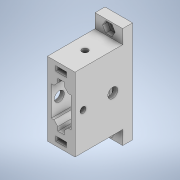
# Autodesk Inventor part: стаканчик_мозговорот
Saved by Autodesk Inventor 2021 (Build 250183000, 183)
## iProperties
Created: 2022-11-16
Part Number: стаканчик_мозговорот
Material: Типовые
Document SubType Name: Modeling
Designer: zmoze
Density: 1 g/cm^3
Appearance: По умолчанию
Author: zmoze
Autodesk Inventor part; units mm, degrees
sketch "Эскиз1" plane through (0, 0, 0) normal (0, 0, 1) x (1, 0, 0)
  line L0 (0, 0) -> (3.3, 0)
  line L1 (3.3, 0) -> (3.3, 15)
  line L2 (3.3, 15) -> (0, 15)
  line L3 (0, 15) -> (0, 0)
  line L4 (3.3, -4) -> (6.6, -4)
  line L5 (6.6, -4) -> (6.6, 19)
  line L6 (6.6, 19) -> (3.3, 19)
  line L7 (3.3, 19) -> (3.3, -4)
  line L8 (6.6, 0) -> (9.9, 0)
  line L9 (9.9, 0) -> (9.9, 15)
  line L10 (9.9, 15) -> (6.6, 15)
  line L11 (6.6, 15) -> (6.6, 0)
  line L12 (-2, 21) -> (11.9, 21)
  line L13 (11.9, 21) -> (11.9, -6)
  line L14 (11.9, -6) -> (-2, -6)
  line L15 (-2, -6) -> (-2, 21)
  dimension "d2" = 15
  dimension "d3" = 23
  dimension "d4" = 4
  dimension "d5" = 3.3
  dimension "d6" = 2
  dimension "d7" = 2
  dimension "d8" = 2
  dimension "d9" = 2
  constraints: 32 end point, 8 parallel, 4 horizontal, 4 perpendicular, 4 point on line, 2 equal length
  measures "d2" distance of L2.end L0.start
  measures "d3" distance of L6.end L4.start
  measures "d4" distance between parallel lines of L2 L6
  measures "d5" distance of L1.end L2.end
  measures "d6" distance between parallel lines of L12 L6
  measures "d7" distance between parallel lines of L3 L15
  measures "d8" distance between parallel lines of L13 L9
  measures "d9" distance between parallel lines of L14 L4
extrude "Выдавливание1" add sketch "Эскиз1" along normal blind 24
sketch "Эскиз2" plane through (0, 0, 0) normal (0, 0, -1) x (-1, 0, 0)
  line L0 (2, 21) -> (2, -6) projected
  line L1 (2, -6) -> (-11.9, -6) projected
  line L2 (2, 21) -> (2, -6) projected
  line L3 (-11.9, 21) -> (2, 21) projected
  line L4 (-11.9, -6) -> (-11.9, 21) projected
  line L5 (0, 0) -> (0, 15) projected
  line L6 (-3.3, 0) -> (0, 0) projected
  line L7 (-3.3, -4) -> (-3.3, 0) projected
  line L8 (-6.6, -4) -> (-3.3, -4) projected
  line L9 (-6.6, 0) -> (-6.6, -4) projected
  line L10 (-9.9, 0) -> (-6.6, 0) projected
  line L11 (-9.9, 15) -> (-9.9, 0) projected
  line L12 (-6.6, 15) -> (-9.9, 15) projected
  line L13 (-6.6, 19) -> (-6.6, 15) projected
  line L14 (-3.3, 19) -> (-6.6, 19) projected
  line L15 (-3.3, 15) -> (-3.3, 19) projected
  line L16 (0, 15) -> (-3.3, 15) projected
  line L17 (-11.9, 21) -> (2, 21) projected
  line L18 (-11.9, 21) -> (2, 21)
  line L19 (2, 21) -> (2, 33)
  line L20 (2, 33) -> (-11.9, 33)
  line L21 (-11.9, 33) -> (-11.9, 21)
  line L22 (-11.9, -6) -> (2, -6)
  line L23 (2, -6) -> (2, -18)
  line L24 (2, -18) -> (-11.9, -18)
  line L25 (-11.9, -18) -> (-11.9, -6)
  point P0 (2, -6)
  dimension "d12" = 12
  constraints: 16 end point, 4 parallel, 2 collinear, 2 horizontal, 2 perpendicular, 1 point on line
  measures "d12" distance of L18.end L19.end
extrude "Выдавливание2" add sketch "Эскиз2" along normal blind 5 contours L0 L1 L4 L3 | L3 L21 L20 L19 | L23 L24 L25 L1 | L6 L7 L8 L9 L10 L11 L12 L13 L14 L15 L16 L5
sketch "Эскиз5" plane through (11.9, 21, 24) normal (1, 0, 0) x (0, -1, 0)
  circle A0 centre (13.5, 4) radius 1.5
  circle A1 centre (13.5, 19) radius 2.5
  line L0 (-12, 24) -> (-12, 24) projected
  line L1 (13.5, 4) -> (13.5, 19) construction
  line L2 (27, 0) -> (0, 0) projected
  line L3 (-12, 24) -> (0, 24) projected
  point P0 (13.5, 0)
  dimension "d24" = 3
  dimension "d25" = 5
  dimension "d26" = 15
  dimension "d48" = 5
  constraints: 2 centre point, 2 end point, 1 midpoint, 1 point on line, 1 vertical
  measures "d24" diameter of A0
  measures "d25" diameter of A1
  measures "d26" distance of L1.end L1.start
  measures "d48" distance from line of L1.end L3
sketch "Эскиз6" plane through (-2, -6, 24) normal (-1, 0, 0) x (0, -1, 0)
  circle A0 centre (-13.5, -4) radius 2.5
  circle A1 centre (-13.5, -19) radius 1.5
  line L0 (-13.5, -4) -> (-13.5, -19) construction
  line L1 (0, 0) -> (0, 0) construction
  line L2 (12, -24) -> (12, -24) construction
  line L3 (-27, 0) -> (0, 0) projected
  line L4 (12, -24) -> (0, -24) projected
  point P0 (-6, -24)
  point P1 (-13.5, 0)
  dimension "d28" = 3
  dimension "d29" = 5
  dimension "d30" = 15
  dimension "d49" = 20
  constraints: 2 centre point, 2 end point, 1 midpoint, 1 point on line, 1 vertical
  measures "d28" diameter of A1
  measures "d29" diameter of A0
  measures "d30" distance of L0.end L0.start
  measures "d49" distance from line of L4 L0.start
extrude "Выдавливание5" cut sketch "Эскиз5" against normal blind 3
extrude "Выдавливание6" cut sketch "Эскиз6" against normal blind 3
ref_plane "РабПлоскость1" through (4.95, -6, 24) normal (-1, 0, 0) x (0, 0, 1)
ref_plane "РабПлоскость2" through (-2, 7.5, 24) normal (0, 1, 0) x (1, 0, 0)
sketch "Эскиз8" plane through (0, 0, 24) normal (0, 0, 1) x (1, 0, 0)
  line L0 (-2, -6) -> (11.9, -6) projected
  line L1 (-2, -18) -> (-2, 33) projected
  line L2 (11.9, -6) -> (-2, -6)
  line L3 (-2, -6) -> (-2, -11)
  line L4 (-2, -11) -> (11.9, -11)
  line L5 (11.9, -11) -> (11.9, -6)
  line L6 (11.9, 33) -> (11.9, 21) projected
  line L7 (11.9, 21) -> (-2, 21)
  line L8 (-2, 21) -> (-2, 26)
  line L9 (-2, 26) -> (11.9, 26)
  line L10 (11.9, 26) -> (11.9, 21)
  point P0 (0, 0)
  point P1 (-2, 21)
  dimension "d38" = 5
  constraints: 16 end point, 4 parallel, 2 horizontal, 2 perpendicular, 2 point on line, 1 collinear
  measures "d38" distance between parallel lines of L0 L4
extrude "Выдавливание8" add sketch "Эскиз8" against normal up to surface (24 mm away)
ref_plane "РабПлоскость3" through (-2, -9, 24) normal (0, -1, 0) x (1, 0, 0)
sketch "Эскиз9" plane through (-2, -9, 24) normal (0, -1, 0) x (1, 0, 0)
  line L0 (0, 0) -> (13.9, 0) projected
  line L1 (9.7, 0) -> (4.2, 0)
  line L2 (4.2, 0) -> (4.2, -22.4123)
  line L3 (4.2, -22.4123) -> (9.7, -22.4123)
  line L4 (9.7, -22.4123) -> (9.7, 0)
  line L5 (9.7, -22.4123) -> (6.95, -24)
  line L6 (6.95, -24) -> (4.2, -22.4123)
  line L7 (4.2, -22.4123) -> (4.2, -19.2369)
  line L8 (4.2, -19.2369) -> (6.95, -17.6491)
  line L9 (6.95, -17.6491) -> (9.7, -19.2369)
  line L10 (9.7, -19.2369) -> (9.7, -22.4123)
  line L11 (5.3, -24) -> (8.6, -24) projected
  point P0 (2, -24)
  point P1 (6.95, -20.8246)
  point P2 (4.2, 0)
  dimension "d42" = 5.5
  constraints: 20 end point, 2 collinear, 2 parallel, 1 horizontal, 1 midpoint, 1 perpendicular, 1 point on line, 13 other
  measures "d42" distance between parallel lines of L2 L4
extrude "Выдавливание9" cut sketch "Эскиз9" against normal blind 2.4
ref_plane "РабПлоскость4" through (-2, 24, 24) normal (0, 1, 0) x (1, 0, 0)
sketch "Эскиз10" plane through (-2, 24, 24) normal (0, 1, 0) x (1, 0, 0)
  line L0 (9.7, 0) -> (9.7, 22.4123) projected
  line L1 (4.2, 22.4123) -> (4.2, 0) projected
  line L2 (9.7, 22.4123) -> (6.95, 24) projected
  line L3 (6.95, 24) -> (4.2, 22.4123) projected
  line L4 (5.3, 0) -> (8.6, 0) projected
  line L5 (8.6, 0) -> (11.9, 0) projected
  line L6 (2, 0) -> (5.3, 0) projected
  point P0 (2, 24)
extrude "Выдавливание10" cut sketch "Эскиз10" against normal blind 2.4
sketch "Эскиз11" plane through (-2, -11, 24) normal (0, -1, 0) x (1, 0, 0)
  line L0 (9.7, -22.4123) -> (9.7, 0) projected
  line L1 (6.95, -24) -> (9.7, -22.4123) projected
  line L2 (4.2, -22.4123) -> (6.95, -24) projected
  line L3 (4.2, 0) -> (4.2, -22.4123) projected
  line L4 (6.95, -24) -> (4.2, -22.4123)
  line L5 (4.2, -22.4123) -> (4.2, -19.2369)
  line L6 (4.2, -19.2369) -> (6.95, -17.6491)
  line L7 (6.95, -17.6491) -> (9.7, -19.2369)
  line L8 (9.7, -19.2369) -> (9.7, -22.4123)
  line L9 (9.7, -22.4123) -> (6.95, -24)
  circle A0 centre (6.95, -20.8246) radius 1.5
  line L10 (13.9, 0) -> (13.9, -24) projected
  line L11 (0, 0) -> (0, -24) projected
  line L12 (0, 0) -> (0, -24) construction
  line L13 (0, -12) -> (13.9, -12) construction
  circle A1 centre (6.95, -12) radius 1.5
  point P0 (2, -24)
  dimension "d50" = 3
  dimension "d57" = 3
  constraints: 14 end point, 3 midpoint, 2 centre point, 1 coincident, 13 other
  measures "d50" diameter of A0
  measures "d57" diameter of A1
extrude "Выдавливание11" cut sketch "Эскиз11" against normal through all contours A1
sketch "Эскиз3" plane through (0, 0, 0) normal (0, 0, 1) x (1, 0, 0)
  circle A0 centre (4.95, 29.5) radius 1.5
  circle A1 centre (4.95, -14.5) radius 1.5
  line L0 (-2, 33) -> (11.9, 33) construction
  line L1 (4.95, 33) -> (4.95, -18) construction
  line L2 (11.9, -18) -> (-2, -18) construction
  point P0 (0, 0)
  dimension "d16" = 3
  dimension "d17" = 3.5
  dimension "d18" = 3.5
  constraints: 2 centre point, 2 end point, 2 midpoint, 2 point on line, 1 equal radius
  measures "d16" diameter of A0
  measures "d17" distance from line of L0 A0.centre
  measures "d18" distance from line of L2 A1.centre
extrude "Выдавливание3" cut sketch "Эскиз3" against normal blind 5
sketch "Эскиз4" plane through (0, 0, 0) normal (0, 0, 1) x (1, 0, 0)
  circle A0 centre (4.95, -14.5) radius 1.5 projected
  circle A1 centre (4.95, 29.5) radius 1.5 projected
  line L0 (4.084, -16) -> (3.2179, -14.5)
  line L1 (3.2179, -14.5) -> (4.084, -13)
  line L2 (4.084, -13) -> (5.816, -13)
  line L3 (5.816, -13) -> (6.6821, -14.5)
  line L4 (6.6821, -14.5) -> (5.816, -16)
  line L5 (5.816, -16) -> (4.084, -16)
  line L6 (4.084, 28) -> (3.2179, 29.5)
  line L7 (3.2179, 29.5) -> (4.084, 31)
  line L8 (4.084, 31) -> (5.816, 31)
  line L9 (5.816, 31) -> (6.6821, 29.5)
  line L10 (6.6821, 29.5) -> (5.816, 28)
  line L11 (5.816, 28) -> (4.084, 28)
  line L12 (3.3623, -11.75) -> (1.7746, -14.5)
  line L13 (1.7746, -14.5) -> (3.3623, -17.25)
  line L14 (3.3623, -17.25) -> (6.5377, -17.25)
  line L15 (6.5377, -17.25) -> (8.1254, -14.5)
  line L16 (8.1254, -14.5) -> (6.5377, -11.75)
  line L17 (6.5377, -11.75) -> (3.3623, -11.75)
  line L18 (3.3623, 32.25) -> (1.7746, 29.5)
  line L19 (1.7746, 29.5) -> (3.3623, 26.75)
  line L20 (3.3623, 26.75) -> (6.5377, 26.75)
  line L21 (6.5377, 26.75) -> (8.1254, 29.5)
  line L22 (8.1254, 29.5) -> (6.5377, 32.25)
  line L23 (6.5377, 32.25) -> (3.3623, 32.25)
  point P0 (0, 0)
  point P1 (4.95, -16)
  point P2 (4.95, 28)
  dimension "d53" = 5.5
  constraints: 48 end point, 2 coincident, 2 horizontal, 2 midpoint, 2 vertical alignment, 1 equal length, 38 other
  measures "d53" distance between parallel lines of L17 L14
extrude "Выдавливание4" cut sketch "Эскиз4" against normal blind 2.5 contours A0 | A0 L3 L4 | A0 L2 L3 | L4 L5 A0 | A0 L1 L2 | L5 L0 A0 | A0 L0 L1 | A1 | A1 L9 L10 | A1 L8 L9 | L10 L11 A1 | A1 L7 L8 | L11 L6 A1 | A1 L6 L7 | L17 L16 L15 L14 L13 L12 | L23 L22 L21 L20 L19 L18
sketch "Эскиз7" plane through (0, 0, 0) normal (0, 0, 1) x (1, 0, 0)
  line L0 (6.6, -4) -> (3.3, -4) projected
  line L1 (3.2528, 19.197) -> (6.6, 19.197)
  line L2 (6.6, 19.197) -> (6.6, -4)
  line L3 (6.6, -4) -> (3.2528, -4)
  line L4 (3.2528, -4) -> (3.2528, 19.197)
  point P0 (0, 0)
  constraints: 8 end point, 2 parallel, 1 horizontal, 1 perpendicular
extrude "Выдавливание7" cut sketch "Эскиз7" against normal blind 2
chamfer "Фаска1" distance 2 angle 45 4 edges at (3.3, 0, 12) (6.6, 0, 12) (3.3, 15, 12) (6.6, 15, 12)
